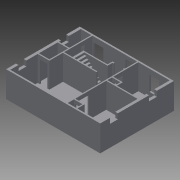
# Autodesk Inventor part: Basement
Saved by Autodesk Inventor 2013 (Build 170138000, 138)
## iProperties
Created: 2013-06-16
Part Number: Basement
Material: Generic
Document SubType Name: Modeling
Designer: Joey
Density: 1 g/cm^3
Author: Joey
Autodesk Inventor part; units mm, degrees
ref_plane "YZ Plane" through (0, 0, 0) normal (1, 0, 0) x (0, 1, 0)
ref_plane "XZ Plane" through (0, 0, 0) normal (0, 1, 0) x (-1, 0, 0)
ref_plane "XY Plane" through (0, 0, 0) normal (0, 0, 1) x (1, 0, 0)
sketch "Sketch1" plane through (0, 0, 0) normal (0, 1, 0) x (-1, 0, 0)
  line L0 (4572, 3671.9134) -> (4572, -3490.8866)
  line L1 (4572, -3490.8866) -> (-4572, -3490.8866)
  line L2 (-4572, -3490.8866) -> (-4572, 3671.9134)
  line L3 (0, 3519.5134) -> (0, 3671.9134)
  line L4 (914.4, 3671.9134) -> (914.4, 3519.5134)
  line L5 (-4318, 1385.9134) -> (-3302, 1385.9134)
  line L6 (-4318, 3519.5134) -> (-3302, 3519.5134)
  line L7 (-3302, 1271.6134) -> (-4318, 1271.6134)
  line L8 (-4318, 1385.9134) -> (-4318, 3519.5134)
  line L9 (-3302, 2757.5134) -> (-3187.7, 2757.5134)
  line L10 (-3187.7, 1843.1134) -> (-3302, 1843.1134)
  line L11 (-4318, 1271.6134) -> (-3302, 1271.6134)
  line L12 (-4318, -557.1866) -> (-4318, 1271.6134)
  line L13 (-3302, 1271.6134) -> (-4318, 1271.6134)
  line L14 (-4318, 1271.6134) -> (-4318, -557.1866)
  line L15 (-3187.7, 763.6134) -> (-3187.7, 1549.4)
  line L16 (1270, 395.3134) -> (4318, 395.3134)
  line L17 (2082.8, -2728.8866) -> (2082.8, -3338.4866)
  line L18 (1270, -2728.8866) -> (1327.15, -2728.8866)
  line L19 (2082.8, -2728.8866) -> (2025.65, -2728.8866)
  line L20 (2025.65, -2728.8866) -> (2025.65, -2614.5866)
  line L21 (2025.65, -2614.5866) -> (2197.1, -2614.5866)
  line L22 (2197.1, -2614.5866) -> (2197.1, -3338.4866)
  line L23 (1327.15, -2728.8866) -> (1327.15, -2614.5866)
  line L24 (1327.15, -2614.5866) -> (1270, -2614.5866)
  line L25 (-3187.7, 3519.5134) -> (-3187.7, 2757.5134)
  line L26 (-3187.7, 1843.1134) -> (-3187.7, 1676.4)
  line L27 (-3302, 1385.9134) -> (-3302, 1843.1134)
  line L28 (-3302, 2757.5134) -> (-3302, 3519.5134)
  line L29 (-4318, -3338.4866) -> (-4318, -671.4866)
  line L30 (1155.7, -2500.2866) -> (1270, -2500.2866)
  line L31 (1155.7, -1281.0866) -> (1270, -1281.0866)
  line L32 (1155.7, -3338.4866) -> (1155.7, -2500.2866)
  line L33 (1155.7, -3338.4866) -> (-4318, -3338.4866)
  line L34 (1270, 395.3134) -> (1270, -1281.0866)
  line L35 (4318, 3519.5134) -> (4318, 509.6134)
  line L36 (4318, 395.3134) -> (4318, -3338.4866)
  line L37 (1270, 3519.5134) -> (4318, 3519.5134)
  line L38 (-3187.7, 649.3134) -> (63.5, 649.3134)
  line L39 (-3187.7, 763.6134) -> (63.5, 763.6134)
  line L40 (63.5, 763.6134) -> (63.5, 649.3134)
  line L41 (-2374.9, 1728.8134) -> (63.5, 1728.8134)
  line L42 (-50.8, 1843.1134) -> (-50.8, 2325.7134)
  line L43 (63.5, 1728.8134) -> (63.5, 2211.4134)
  line L44 (63.5, 2211.4134) -> (165.1, 2211.4134)
  line L45 (-50.8, 2325.7134) -> (165.1, 2325.7134)
  line L46 (2082.8, 509.6134) -> (2082.8, 966.8134)
  line L47 (2082.8, 966.8134) -> (2025.65, 966.8134)
  line L48 (1327.15, 966.8134) -> (1270, 966.8134)
  line L49 (2025.65, 966.8134) -> (2025.65, 1081.1134)
  line L50 (2025.65, 1081.1134) -> (2197.1, 1081.1134)
  line L51 (2197.1, 1081.1134) -> (2197.1, 509.6134)
  line L52 (1270, 966.8134) -> (1270, 509.6134)
  line L53 (-4318, 3519.5134) -> (-3302, 3519.5134)
  line L54 (1155.7, 1995.5134) -> (1270, 1995.5134)
  line L55 (1270, 3519.5134) -> (1270, 1995.5134)
  line L56 (1155.7, -1281.0866) -> (1155.7, 1081.1134)
  line L57 (-3187.7, 3519.5134) -> (0, 3519.5134)
  line L58 (914.4, 3519.5134) -> (1155.7, 3519.5134)
  line L59 (-4572, 3671.9134) -> (0, 3671.9134)
  line L60 (914.4, 3671.9134) -> (4572, 3671.9134)
  line L61 (-4318, -557.1866) -> (-4318, 1271.6134)
  line L62 (-4318, 1385.9134) -> (-4318, 3519.5134)
  line L63 (4318, -3338.4866) -> (2197.1, -3338.4866)
  line L64 (2082.8, -3338.4866) -> (1270, -3338.4866)
  line L65 (1270, 509.6134) -> (2082.8, 509.6134)
  line L66 (2197.1, 509.6134) -> (4318, 509.6134)
  line L67 (1270, -2500.2866) -> (1270, -2614.5866)
  line L68 (1270, -2728.8866) -> (1270, -3338.4866)
  line L69 (1155.7, 1081.1134) -> (1327.15, 1081.1134)
  line L70 (1327.15, 1081.1134) -> (1327.15, 966.8134)
  line L71 (-4318, -557.1866) -> (-3302, -557.1866)
  line L72 (-3302, 3519.5134) -> (-3302, 2757.5134)
  line L73 (-3302, 3519.5134) -> (-4318, 3519.5134)
  line L74 (-3187.7, 2757.5134) -> (-3302, 2757.5134)
  line L75 (-3302, 2757.5134) -> (-3302, 3519.5134)
  line L76 (-3302, 3519.5134) -> (-4318, 3519.5134)
  line L77 (-4318, 3519.5134) -> (-4318, 1385.9134)
  line L78 (-4318, 1271.6134) -> (-4318, -557.1866)
  line L79 (-4318, 1385.9134) -> (-3302, 1385.9134)
  line L80 (-3302, 1271.6134) -> (-4318, 1271.6134)
  line L81 (-4318, 3519.5134) -> (-3302, 3519.5134)
  line L82 (-3302, 1385.9134) -> (-4318, 1385.9134)
  line L83 (-4318, 1385.9134) -> (-4318, 3519.5134)
  line L84 (-3302, 3519.5134) -> (-3302, 2757.5134)
  line L85 (-3302, 1843.1134) -> (-3302, 1385.9134)
  line L86 (-3187.7, 2757.5134) -> (-3302, 2757.5134)
  line L87 (-3302, 2757.5134) -> (-3302, 3519.5134)
  line L88 (-2641.6, 3671.9134) -> (-2527.3, 3671.9134)
  line L89 (-3187.7, 3519.5134) -> (-3187.7, 2757.5134)
  line L90 (-3187.7, 1551.0134) -> (-3187.7, 763.6134)
  line L91 (-2374.9, 1728.8134) -> (63.5, 1728.8134)
  line L92 (63.5, 763.6134) -> (-3187.7, 763.6134)
  line L93 (-3187.7, 763.6134) -> (-3187.7, 1551.0134)
  line L94 (165.1, 2211.4134) -> (165.1, 2325.7134)
  line L95 (1155.7, 2325.7134) -> (1079.5, 2325.7134)
  line L96 (1079.5, 2325.7134) -> (1079.5, 2211.4134)
  line L97 (1079.5, 2211.4134) -> (1155.7, 2211.4134)
  line L98 (1155.7, 1995.5134) -> (1155.7, 2211.4134)
  line L99 (1155.7, 2325.7134) -> (1155.7, 3519.5134)
  line L100 (-3187.7, 1676.4) -> (-3187.7, 1271.6134)
  line L101 (-50.8, 1843.1134) -> (-2374.9, 1843.1134)
  line L102 (-3187.7, 1665.3134) -> (-3187.7, 1551.0134)
  line L103 (-4318, -671.4866) -> (-3352.8, -671.4866)
  line L104 (-3302, 1271.6134) -> (-3302, -557.1866)
  line L105 (-3352.8, -671.4866) -> (-3187.7, -671.4866)
  line L106 (-2374.9, 1843.1134) -> (-2374.9, 763.6134)
  line L107 (-3187.7, -671.4866) -> (-3187.7, 649.3134)
  line L108 (-3187.7, 649.3134) -> (-3187.7, 596.9)
  line L109 (-3187.7, 1271.6134) -> (-3187.7, 763.6134)
  line L110 (-3187.7, 649.3134) -> (-3187.7, 596.9)
  point P0 (0, 0)
  dimension "d0" = 9144
  dimension "d8" = 3657.6
  dimension "d9" = 4572
  dimension "d13" = 114.3
  dimension "d56" = 254
  dimension "d59" = 114.3
  dimension "d60" = 965.2
  dimension "d85" = 2133.6
  dimension "d94" = 3048
  dimension "d95" = 114.3
  dimension "d96" = 114.3
  dimension "d98" = 152.4
  dimension "d148" = 152.4
  dimension "d149" = 254
  dimension "d150" = 254
  dimension "d151" = 254
  dimension "d152" = 254
  dimension "d153" = 152.4
  dimension "d154" = 152.4
  dimension "d155" = 7162.8
  dimension "d156" = 3048
  dimension "d157" = 114.3
  dimension "d160" = 152.4
  dimension "d161" = 152.4
  dimension "d163" = 114.3
  dimension "d167" = 3733.8
  dimension "d168" = 3009.9
  dimension "d169" = 3009.9
  dimension "d171" = 698.5
  dimension "d172" = 57.15
  dimension "d173" = 114.3
  dimension "d174" = 152.4
  dimension "d175" = 114.3
  dimension "d176" = 114.3
  dimension "d177" = 609.6
  dimension "d178" = 609.6
  dimension "d179" = 1219.2
  dimension "d180" = 114.3
  dimension "d181" = 114.3
  dimension "d182" = 457.2
  dimension "d184" = 457.2
  dimension "d188" = 698.5
  dimension "d189" = 57.15
  dimension "d190" = 57.15
  dimension "d191" = 114.3
  dimension "d192" = 57.15
  dimension "d195" = 1016
  dimension "d196" = 114.3
  dimension "d197" = 114.3
  dimension "d198" = 1016
  dimension "d199" = 914.4
  dimension "d200" = 762
  dimension "d217" = 114.3
  dimension "d289" = 914.4
  dimension "d290" = 114.3
  dimension "d291" = 482.6
  dimension "d292" = 76.2
  dimension "d293" = 114.3
  dimension "d296" = 114.3
  dimension "d297" = 1828.8
  dimension "d299" = 114.3
  dimension "d302" = 3251.2
  dimension "d303" = 2438.4
  dimension "d304" = 101.6
  constraints: 222 end point, 88 perpendicular, 53 parallel, 15 collinear, 14 horizontal, 4 point on line
  measures "d0" distance between parallel lines of L0 L2
  measures "d8" distance between parallel lines of L0 L4
  measures "d9" distance between parallel lines of L2 L3
  measures "d13" distance between parallel lines of L5 L7
  measures "d56" distance between parallel lines of L0 L35
  measures "d59" distance of L39.end L38.end
  measures "d60" distance between parallel lines of L39 L41
  measures "d85" distance between parallel lines of L5 L6
  measures "d94" distance between parallel lines of L35 L55
  measures "d95" distance between parallel lines of L43 L42
  measures "d96" distance between parallel lines of L27 L26
  measures "d98" distance between parallel lines of L1 L64
  measures "d148" distance between parallel lines of L1 L63
  measures "d149" distance between parallel lines of L0 L36
  measures "d150" distance between parallel lines of L2 L29
  measures "d151" distance between parallel lines of L2 L12
  measures "d152" distance between parallel lines of L2 L8
  measures "d153" distance between parallel lines of L59 L6
  measures "d154" distance between parallel lines of L60 L58
  measures "d155" distance between parallel lines of L1 L60
  measures "d156" distance between parallel lines of L36 L34
  measures "d157" distance between parallel lines of L56 L52
  measures "d160" distance between parallel lines of L60 L37
  measures "d161" distance between parallel lines of L59 L57
  measures "d163" distance between parallel lines of L25 L28
  measures "d167" distance between parallel lines of L16 L63
  measures "d168" distance between parallel lines of L37 L66
  measures "d169" distance between parallel lines of L37 L65
  measures "d171" distance between parallel lines of L20 L23
  measures "d172" distance between parallel lines of L20 L17
  measures "d173" distance between parallel lines of L22 L17
  measures "d174" distance between parallel lines of L1 L33
  measures "d175" distance between parallel lines of L21 L19
  measures "d176" distance between parallel lines of L24 L18
  measures "d177" distance between parallel lines of L64 L18
  measures "d178" distance between parallel lines of L64 L19
  measures "d179" distance between parallel lines of L30 L31
  measures "d180" distance between parallel lines of L30 L24
  measures "d181" distance between parallel lines of L32 L68
  measures "d182" distance between parallel lines of L65 L47
  measures "d184" distance between parallel lines of L65 L48
  measures "d188" distance between parallel lines of L49 L70
  measures "d189" distance between parallel lines of L52 L70
  measures "d190" distance between parallel lines of L46 L49
  measures "d191" distance between parallel lines of L51 L46
  measures "d192" distance between parallel lines of L68 L23
  measures "d195" distance between parallel lines of L8 L27
  measures "d196" distance between parallel lines of L48 L69
  measures "d197" distance between parallel lines of L47 L50
  measures "d198" distance between parallel lines of L8 L28
  measures "d199" distance from line of L9.start L10
  measures "d200" distance between parallel lines of L9 L57
  measures "d217" distance between parallel lines of L32 L67
  measures "d289" distance between parallel lines of L69 L54
  measures "d290" distance between parallel lines of L99 L55
  measures "d291" distance between parallel lines of L45 L101
  measures "d292" distance between parallel lines of L99 L96
  measures "d293" distance between parallel lines of L41 L101
  measures "d296" distance between parallel lines of L103 L71
  measures "d297" distance between parallel lines of L7 L71
  measures "d299" distance between parallel lines of L56 L34
  measures "d302" distance between parallel lines of L15 L43
  measures "d303" distance between parallel lines of L43 L106
  measures "d304" distance between parallel lines of L94 L43
extrude "Extrusion8" add sketch "Sketch1" along normal blind 2438.4 contours L0 L1 L2 L59 L3 L57 L25 L9 L28 L6 L8 L5 L27 L10 L26 L100 L90 L15 L39 L40 L38 L107 L105 L103 L29 L33 L32 L30 L67 L24 L23 L18 L68 L64 L17 L19 L20 L21 L22 L63 L36 L16 L34 L31 L56 L69 L70 L48 L52 L65 L46 L47 L49 L50 L51 L66 L35 L37 L55 L54 L98 L97 L96 L95 L99 L58 L4 L60 | L104 L71 L12 L7
sketch "Sketch8" plane through (0, 0, 0) normal (0, -1, 0) x (1, 0, 0)
  line L0 (-4572, 3671.9134) -> (4572, 3671.9134)
  line L1 (4572, 3671.9134) -> (4572, -3490.8866)
  line L2 (4572, -3490.8866) -> (-4572, -3490.8866)
  line L3 (-4572, -3490.8866) -> (-4572, 3671.9134)
  point P0 (0, 0)
  constraints: 8 end point, 2 parallel, 1 horizontal, 1 perpendicular
extrude "Extrusion9" add sketch "Sketch8" along normal blind 76.2
sketch "Sketch11" plane through (-4572, 2438.4, -3490.8866) normal (-1, 0, 0) x (0, 0, 1)
  line L0 (7162.8, -2514.6) -> (7162.8, 0) projected
  line L1 (0, 0) -> (7162.8, 0) projected
  line L2 (0, -2514.6) -> (0, 0) projected
  line L3 (952.5, 0) -> (1714.5, 0)
  line L4 (1714.5, 0) -> (1714.5, -508)
  line L5 (1714.5, -508) -> (952.5, -508)
  line L6 (952.5, -508) -> (952.5, 0)
  line L7 (4749.8, 0) -> (5511.8, 0)
  line L8 (5511.8, 0) -> (5511.8, -508)
  line L9 (5511.8, -508) -> (4749.8, -508)
  line L10 (4749.8, -508) -> (4749.8, 0)
  point P0 (3490.8866, -2438.4)
  dimension "d258" = 762
  dimension "d260" = 508
  dimension "d261" = 952.5
  dimension "d262" = 762
  dimension "d263" = 508
  dimension "d264" = 1651
  constraints: 16 end point, 4 parallel, 2 horizontal, 2 perpendicular, 2 point on line
  measures "d258" distance of L4.end L5.end
  measures "d260" distance of L3.end L4.end
  measures "d261" distance between parallel lines of L2 L6
  measures "d262" distance of L8.end L9.end
  measures "d263" distance between parallel lines of L9 L1
  measures "d264" distance between parallel lines of L0 L8
extrude "Extrusion12" cut sketch "Sketch11" against normal blind 254
sketch "Sketch12" plane through (4572, 2438.4, 3671.9134) normal (1, 0, 0) x (0, 0, -1)
  line L0 (7162.8, -2514.6) -> (7162.8, 0) projected
  line L1 (0, 0) -> (7162.8, 0) projected
  line L2 (0, 0) -> (0, -2514.6) projected
  line L3 (1320.8, 0) -> (2082.8, 0)
  line L4 (2082.8, 0) -> (2082.8, -508)
  line L5 (2082.8, -508) -> (1320.8, -508)
  line L6 (1320.8, -508) -> (1320.8, 0)
  line L7 (5448.3, 0) -> (6210.3, 0)
  line L8 (6210.3, 0) -> (6210.3, -508)
  line L9 (6210.3, -508) -> (5448.3, -508)
  line L10 (5448.3, -508) -> (5448.3, 0)
  point P0 (3671.9134, -2438.4)
  dimension "d267" = 508
  dimension "d268" = 762
  dimension "d269" = 1320.8
  dimension "d270" = 952.5
  dimension "d271" = 762
  dimension "d272" = 508
  constraints: 16 end point, 4 parallel, 2 horizontal, 2 perpendicular, 2 point on line
  measures "d267" distance between parallel lines of L5 L1
  measures "d268" distance between parallel lines of L6 L4
  measures "d269" distance between parallel lines of L2 L6
  measures "d270" distance between parallel lines of L0 L8
  measures "d271" distance between parallel lines of L10 L8
  measures "d272" distance between parallel lines of L9 L1
extrude "Extrusion13" cut sketch "Sketch12" against normal blind 254
sketch "Sketch13" plane through (-4572, 2438.4, 3671.9134) normal (0, 0, 1) x (1, 0, 0)
  line L0 (0, 0) -> (9144, 0) projected
  line L1 (0, -2514.6) -> (0, 0) projected
  line L2 (9144, 0) -> (9144, -2514.6) projected
  line L3 (6705.6, -508) -> (7670.8, -508)
  line L4 (7670.8, -508) -> (7670.8, -1955.8)
  line L5 (7670.8, -1955.8) -> (6705.6, -1955.8)
  line L6 (6705.6, -1955.8) -> (6705.6, -508)
  line L7 (1257.3, -508) -> (2222.5, -508)
  line L8 (2222.5, -508) -> (2222.5, -1955.8)
  line L9 (2222.5, -1955.8) -> (1257.3, -1955.8)
  line L10 (1257.3, -1955.8) -> (1257.3, -508)
  dimension "d275" = 1447.8
  dimension "d277" = 965.2
  dimension "d278" = 1473.2
  dimension "d279" = 508
  dimension "d280" = 508
  dimension "d281" = 1257.3
  dimension "d282" = 965.2
  dimension "d283" = 1447.8
  constraints: 16 end point, 4 parallel, 2 horizontal, 2 perpendicular
  measures "d275" distance between parallel lines of L5 L3
  measures "d277" distance of L4.end L5.end
  measures "d278" distance between parallel lines of L2 L4
  measures "d279" distance between parallel lines of L0 L3
  measures "d280" distance between parallel lines of L0 L7
  measures "d281" distance between parallel lines of L1 L10
  measures "d282" distance between parallel lines of L8 L10
  measures "d283" distance between parallel lines of L9 L7
extrude "Extrusion14" cut sketch "Sketch13" against normal blind 254
extrude "Extrusion15" add sketch "Sketch1" along normal blind 2438.4 contours L106 L101 L42 L45 L94 L44 L43 L41
extrude "Extrusion16" cut sketch "Sketch1" along normal blind 2438.4 contours L104 L71 L12 L7
sketch "Sketch14" plane through (0, 2438.4, 0) normal (0, 1, 0) x (1, 0, 0)
  line L0 (2374.9, -1728.8134) -> (2374.9, -1843.1134) projected
  line L1 (2374.9, -1843.1134) -> (50.8, -1843.1134) projected
  line L2 (50.8, -1843.1134) -> (50.8, -2325.7134) projected
  line L3 (50.8, -2325.7134) -> (-165.1, -2325.7134) projected
  line L4 (-165.1, -2325.7134) -> (-165.1, -2211.4134) projected
  line L5 (-165.1, -2211.4134) -> (-63.5, -2211.4134) projected
  line L6 (-63.5, -2211.4134) -> (-63.5, -1728.8134) projected
  line L7 (-63.5, -1728.8134) -> (2374.9, -1728.8134) projected
  line L8 (-914.4, -3671.9134) -> (-914.4, -3519.5134) projected
  line L9 (0, -3671.9134) -> (-914.4, -3671.9134) projected
  line L10 (0, -3519.5134) -> (0, -3671.9134) projected
  line L11 (3187.7, -3519.5134) -> (0, -3519.5134) projected
  line L12 (3187.7, -2757.5134) -> (3187.7, -3519.5134) projected
  line L13 (3302, -2757.5134) -> (3187.7, -2757.5134) projected
  line L14 (3302, -3519.5134) -> (3302, -2757.5134) projected
  line L15 (4318, -3519.5134) -> (3302, -3519.5134) projected
  line L16 (4318, -1385.9134) -> (4318, -3519.5134) projected
  line L17 (3302, -1385.9134) -> (4318, -1385.9134) projected
  line L18 (3302, -1843.1134) -> (3302, -1385.9134) projected
  line L19 (3187.7, -1843.1134) -> (3302, -1843.1134) projected
  line L20 (3187.7, -763.6134) -> (3187.7, -1843.1134) projected
  line L21 (-63.5, -763.6134) -> (3187.7, -763.6134) projected
  line L22 (-63.5, -649.3134) -> (-63.5, -763.6134) projected
  line L23 (3187.7, -649.3134) -> (-63.5, -649.3134) projected
  line L24 (3187.7, 671.4866) -> (3187.7, -649.3134) projected
  line L25 (4318, 671.4866) -> (3187.7, 671.4866) projected
  line L26 (4318, 3338.4866) -> (4318, 671.4866) projected
  line L27 (-1155.7, 3338.4866) -> (4318, 3338.4866) projected
  line L28 (-1155.7, 2500.2866) -> (-1155.7, 3338.4866) projected
  line L29 (-1270, 2500.2866) -> (-1155.7, 2500.2866) projected
  line L30 (-1270, 2614.5866) -> (-1270, 2500.2866) projected
  line L31 (-1327.15, 2614.5866) -> (-1270, 2614.5866) projected
  line L32 (-1327.15, 2728.8866) -> (-1327.15, 2614.5866) projected
  line L33 (-1270, 2728.8866) -> (-1327.15, 2728.8866) projected
  line L34 (-1270, 3338.4866) -> (-1270, 2728.8866) projected
  line L35 (-2082.8, 3338.4866) -> (-1270, 3338.4866) projected
  line L36 (-2082.8, 2728.8866) -> (-2082.8, 3338.4866) projected
  line L37 (-2025.65, 2728.8866) -> (-2082.8, 2728.8866) projected
  line L38 (-2025.65, 2614.5866) -> (-2025.65, 2728.8866) projected
  line L39 (-2197.1, 2614.5866) -> (-2025.65, 2614.5866) projected
  line L40 (-2197.1, 3338.4866) -> (-2197.1, 2614.5866) projected
  line L41 (-4318, 3338.4866) -> (-2197.1, 3338.4866) projected
  line L42 (-4318, -395.3134) -> (-4318, 3338.4866) projected
  line L43 (-1270, -395.3134) -> (-4318, -395.3134) projected
  line L44 (-1270, 1281.0866) -> (-1270, -395.3134) projected
  line L45 (-1155.7, 1281.0866) -> (-1270, 1281.0866) projected
  line L46 (-1155.7, -1081.1134) -> (-1155.7, 1281.0866) projected
  line L47 (-1327.15, -1081.1134) -> (-1155.7, -1081.1134) projected
  line L48 (-1327.15, -966.8134) -> (-1327.15, -1081.1134) projected
  line L49 (-1270, -966.8134) -> (-1327.15, -966.8134) projected
  line L50 (-1270, -509.6134) -> (-1270, -966.8134) projected
  line L51 (-2082.8, -509.6134) -> (-1270, -509.6134) projected
  line L52 (-2082.8, -966.8134) -> (-2082.8, -509.6134) projected
  line L53 (-2025.65, -966.8134) -> (-2082.8, -966.8134) projected
  line L54 (-2025.65, -1081.1134) -> (-2025.65, -966.8134) projected
  line L55 (-2197.1, -1081.1134) -> (-2025.65, -1081.1134) projected
  line L56 (-2197.1, -509.6134) -> (-2197.1, -1081.1134) projected
  line L57 (-4318, -509.6134) -> (-2197.1, -509.6134) projected
  line L58 (-4318, -3519.5134) -> (-4318, -509.6134) projected
  line L59 (-1270, -3519.5134) -> (-4318, -3519.5134) projected
  line L60 (-1270, -1995.5134) -> (-1270, -3519.5134) projected
  line L61 (-1155.7, -1995.5134) -> (-1270, -1995.5134) projected
  line L62 (-1155.7, -2211.4134) -> (-1155.7, -1995.5134) projected
  line L63 (-1079.5, -2211.4134) -> (-1155.7, -2211.4134) projected
  line L64 (-1079.5, -2325.7134) -> (-1079.5, -2211.4134) projected
  line L65 (-1155.7, -2325.7134) -> (-1079.5, -2325.7134) projected
  line L66 (-1155.7, -3519.5134) -> (-1155.7, -2325.7134) projected
  line L67 (-914.4, -3519.5134) -> (-1155.7, -3519.5134) projected
  line L68 (-2025.65, 2728.8866) -> (-1327.15, 2728.8866)
  line L69 (-1327.15, 2728.8866) -> (-1327.15, 2614.5866)
  line L70 (-1327.15, 2614.5866) -> (-2025.65, 2614.5866)
  line L71 (-2025.65, 2614.5866) -> (-2025.65, 2728.8866)
  line L72 (-1270, 2500.2866) -> (-1155.7, 2500.2866)
  line L73 (-1155.7, 2500.2866) -> (-1155.7, 1281.0866)
  line L74 (-1155.7, 1281.0866) -> (-1270, 1281.0866)
  line L75 (-1270, 1281.0866) -> (-1270, 2500.2866)
  line L76 (-1327.15, -1081.1134) -> (-2025.65, -1081.1134)
  line L77 (-2025.65, -1081.1134) -> (-2025.65, -966.8134)
  line L78 (-2025.65, -966.8134) -> (-1327.15, -966.8134)
  line L79 (-1327.15, -966.8134) -> (-1327.15, -1081.1134)
  line L80 (3302, -1843.1134) -> (3187.7, -1843.1134)
  line L81 (3187.7, -1843.1134) -> (3187.7, -2757.5134)
  line L82 (3187.7, -2757.5134) -> (3302, -2757.5134)
  line L83 (3302, -2757.5134) -> (3302, -1843.1134)
  line L84 (-165.1, -2211.4134) -> (-165.1, -2325.7134)
  line L85 (-1079.5, -2325.7134) -> (-1079.5, -2211.4134)
  line L86 (-914.4, -3519.5134) -> (0, -3519.5134)
  line L87 (0, -3519.5134) -> (0, -3671.9134)
  line L88 (0, -3671.9134) -> (-914.4, -3671.9134)
  line L89 (-914.4, -3671.9134) -> (-914.4, -3519.5134)
  line L90 (-1270, -1995.5134) -> (-1155.7, -1995.5134)
  line L91 (-1155.7, -1995.5134) -> (-1155.7, -1081.1134)
  line L92 (-1155.7, -1081.1134) -> (-1270, -1081.1134)
  line L93 (-1270, -1081.1134) -> (-1270, -1995.5134)
  point P0 (0, 0)
  constraints: 52 end point, 13 parallel, 6 horizontal, 6 perpendicular
sketch "Sketch15" plane through (4318, 2438.4, -671.4866) normal (0, 0, -1) x (-1, 0, 0)
  line L0 (0, -2438.4) -> (1130.3, -2438.4) projected
  line L1 (1130.3, -2438.4) -> (1130.3, 0) projected
  line L2 (0, 0) -> (1130.3, 0) projected
  line L3 (209.55, -2438.4) -> (920.75, -2438.4)
  line L4 (920.75, -2438.4) -> (920.75, -355.6)
  line L5 (920.75, -355.6) -> (209.55, -355.6)
  line L6 (209.55, -355.6) -> (209.55, -2438.4)
  point P0 (4318, -2438.4)
  dimension "d311" = 711.2
  dimension "d313" = 209.55
  dimension "d314" = 355.6
  constraints: 8 end point, 2 parallel, 1 horizontal, 1 perpendicular, 1 point on line
  measures "d311" distance between parallel lines of L4 L6
  measures "d313" distance between parallel lines of L1 L4
  measures "d314" distance between parallel lines of L2 L5
sketch "Sketch16" plane through (2374.9, 0, 1728.8134) normal (0, 0, -1) x (-1, 0, 0)
  line L0 (2438.4, 0) -> (0, 0) projected
  line L1 (0, 2438.4) -> (203.2, 2438.4)
  line L2 (203.2, 2438.4) -> (203.2, 2235.2)
  line L3 (203.2, 2235.2) -> (0, 2235.2)
  line L4 (0, 2235.2) -> (0, 2438.4)
  line L5 (203.2, 2235.2) -> (406.4, 2235.2)
  line L6 (406.4, 2235.2) -> (406.4, 2032)
  line L7 (406.4, 2032) -> (203.2, 2032)
  line L8 (203.2, 2032) -> (203.2, 2235.2)
  line L9 (406.4, 2032) -> (609.6, 2032)
  line L10 (609.6, 2032) -> (609.6, 1828.8)
  line L11 (609.6, 1828.8) -> (406.4, 1828.8)
  line L12 (406.4, 1828.8) -> (406.4, 2032)
  line L13 (609.6, 1828.8) -> (812.8, 1828.8)
  line L14 (812.8, 1828.8) -> (812.8, 1625.6)
  line L15 (812.8, 1625.6) -> (609.6, 1625.6)
  line L16 (609.6, 1625.6) -> (609.6, 1828.8)
  line L17 (812.8, 1625.6) -> (1016, 1625.6)
  line L18 (1016, 1625.6) -> (1016, 1422.4)
  line L19 (1016, 1422.4) -> (812.8, 1422.4)
  line L20 (812.8, 1422.4) -> (812.8, 1625.6)
  line L21 (1016, 1422.4) -> (1219.2, 1422.4)
  line L22 (1219.2, 1422.4) -> (1219.2, 1219.2)
  line L23 (1219.2, 1219.2) -> (1016, 1219.2)
  line L24 (1016, 1219.2) -> (1016, 1422.4)
  line L25 (1219.2, 1219.2) -> (1422.4, 1219.2)
  line L26 (1422.4, 1219.2) -> (1422.4, 1016)
  line L27 (1422.4, 1016) -> (1219.2, 1016)
  line L28 (1219.2, 1016) -> (1219.2, 1219.2)
  line L29 (1422.4, 1016) -> (1625.6, 1016)
  line L30 (1625.6, 1016) -> (1625.6, 812.8)
  line L31 (1625.6, 812.8) -> (1422.4, 812.8)
  line L32 (1422.4, 812.8) -> (1422.4, 1016)
  line L33 (1625.6, 812.8) -> (1828.8, 812.8)
  line L34 (1828.8, 812.8) -> (1828.8, 609.6)
  line L35 (1828.8, 609.6) -> (1625.6, 609.6)
  line L36 (1625.6, 609.6) -> (1625.6, 812.8)
  line L37 (1828.8, 609.6) -> (2032, 609.6)
  line L38 (2032, 609.6) -> (2032, 406.4)
  line L39 (2032, 406.4) -> (1828.8, 406.4)
  line L40 (1828.8, 406.4) -> (1828.8, 609.6)
  line L41 (2032, 406.4) -> (2235.2, 406.4)
  line L42 (2235.2, 406.4) -> (2235.2, 203.2)
  line L43 (2235.2, 203.2) -> (2032, 203.2)
  line L44 (2032, 203.2) -> (2032, 406.4)
  line L45 (2235.2, 203.2) -> (2438.4, 203.2)
  line L46 (2438.4, 203.2) -> (2438.4, 0)
  line L47 (2438.4, 0) -> (2235.2, 0)
  line L48 (2235.2, 0) -> (2235.2, 203.2)
  line L49 (0, 2438.4) -> (2438.4, 0)
  point P0 (2374.9, 0)
  dimension "d317" = 203.2
  dimension "d319" = 203.2
  dimension "d320" = 203.2
  dimension "d321" = 203.2
  dimension "d322" = 203.2
  dimension "d323" = 203.2
  dimension "d324" = 203.2
  dimension "d325" = 203.2
  dimension "d326" = 203.2
  dimension "d327" = 203.2
  dimension "d328" = 203.2
  dimension "d329" = 203.2
  dimension "d330" = 203.2
  dimension "d331" = 203.2
  dimension "d332" = 203.2
  dimension "d333" = 203.2
  dimension "d334" = 203.2
  dimension "d335" = 203.2
  dimension "d336" = 203.2
  dimension "d337" = 203.2
  dimension "d338" = 203.2
  dimension "d339" = 203.2
  constraints: 98 end point, 24 parallel, 12 horizontal, 12 perpendicular
  measures "d317" distance of L2.end L3.end
  measures "d319" distance of L6.end L7.end
  measures "d320" distance of L10.end L11.end
  measures "d321" distance of L14.end L15.end
  measures "d322" distance of L18.end L19.end
  measures "d323" distance of L22.end L23.end
  measures "d324" distance of L26.end L27.end
  measures "d325" distance of L30.end L31.end
  measures "d326" distance of L34.end L35.end
  measures "d327" distance of L38.end L39.end
  measures "d328" distance of L42.end L43.end
  measures "d329" distance between parallel lines of L0 L45
  measures "d330" distance between parallel lines of L43 L41
  measures "d331" distance between parallel lines of L39 L37
  measures "d332" distance between parallel lines of L35 L33
  measures "d333" distance between parallel lines of L31 L29
  measures "d334" distance between parallel lines of L27 L25
  measures "d335" distance between parallel lines of L21 L23
  measures "d336" distance between parallel lines of L17 L19
  measures "d337" distance between parallel lines of L15 L13
  measures "d338" distance between parallel lines of L11 L9
  measures "d339" distance between parallel lines of L7 L5
extrude "Extrusion20" add sketch "Sketch14" against normal blind 355.6 contours L8 L86 L10 L9 | L81 L19 L83 L13 | L61 L93 L47 L91 | L45 L75 L29 L73 | L76 L54 L78 L48 | L70 L38 L68 L32
extrude "Extrusion21" add sketch "Sketch16" along normal blind 965.2
extrude "Extrusion22" cut sketch "Sketch15" against normal blind 114.3
body "Solid2"
